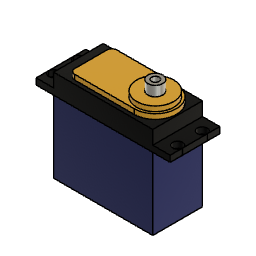
标准舵机 v4 (Autodesk Fusion 360 design; units mm, degrees)
Autodesk Fusion 360 part; units mm, degrees
note: some values were not read from the file. Set by a fixed rule: which sketch regions a step uses.
sketch "草图1" plane through (0, 0, 0) normal (0, 0, 1) x (1, 0, 0)
  line L0 (0, 0) -> (40, 0)
  line L1 (40, 0) -> (40, 20)
  line L2 (40, 20) -> (0, 20)
  line L3 (0, 20) -> (0, 0)
  dimension "d1" = 40
  dimension "d2" = 20
  constraint horizontal L0
  constraint vertical L1
  constraint horizontal L2
  constraint vertical L3
  constraint coincident L0.start L3.end
  measures "d1" distance of L0.start L0.end
  measures "d2" distance of L0.start L2.end
extrude "拉伸1" add sketch "草图1" along normal blind 29 makes body 1
sketch "草图2" plane through (0, 0, 29) normal (0, 0, 1) x (-1, 0, 0)
  line L0 (0, -20) -> (0, 0)
  line L1 (0, 0) -> (-40, 0)
  line L2 (-40, 0) -> (-40, -20)
  line L3 (-40, -20) -> (0, -20)
  line L4 (7, -20) -> (-47, -20)
  line L5 (-47, -20) -> (-47, 0)
  line L6 (-47, 0) -> (7, 0)
  line L7 (7, 0) -> (7, -20)
  line L8 (-20, -21.776) -> (-20, 15.224)
  line L9 (-62, -9.9999) -> (-62, -10)
  line L10 (-62, -10) -> (12.0034, -10)
  line L11 (12.0034, -10) -> (12.0034, -9.9999)
  circle A0 centre (5, -15) radius 2
  circle A1 centre (-45, -15) radius 2
  circle A2 centre (5, -5) radius 2
  circle A3 centre (-45, -5) radius 2
  dimension "d5" = 54
  dimension "d6" = 20
  dimension "d7" = 4
  dimension "d8" = 50
  dimension "d9" = 10
  constraint horizontal L4
  constraint vertical L5
  constraint horizontal L6
  constraint vertical L7
  constraint vertical L8
  constraint symmetric L0 L2 L8
  constraint symmetric L5 L7 L8
  constraint coincident L0.end L6
  constraint horizontal L10
  constraint symmetric L8 A0 A1
  constraint symmetric L10 A0 A2
  constraint symmetric L10 A1 A3
  constraint symmetric L4 L6 L10
  measures "d5" distance of L4.start L4.end
  measures "d6" distance of L4.start L6.end
  measures "d7" diameter of A0
  measures "d8" distance of A0.centre A1.centre
  measures "d9" distance of A0.centre A2.centre
extrude "拉伸2" add sketch "草图2" 1 faces at (13.3333, 13.3333, 29) along normal blind 2.5 separate body on bodies 1 makes body 2
sketch "草图3" plane through (0, 0, 31.5) normal (0, 0, 1) x (-1, 0, 0)
  line L0 (-47, -20) -> (7, -20)
  line L1 (7, -20) -> (7, -15)
  circle A0 centre (5, -15) radius 2
  line L2 (7, -15) -> (7, -5)
  circle A1 centre (5, -5) radius 2
  line L3 (7, -5) -> (7, 0)
  line L4 (7, 0) -> (-47, 0)
  line L5 (-47, 0) -> (-47, -5)
  circle A2 centre (-45, -5) radius 2
  line L6 (-47, -5) -> (-47, -15)
  circle A3 centre (-45, -15) radius 2
  line L7 (-47, -15) -> (-47, -20)
  line L8 (0, 0) -> (-40, 0)
  line L9 (-40, 0) -> (-40, -20)
  line L10 (-40, -20) -> (0, -20)
  line L11 (0, -20) -> (0, 0)
  dimension "d12" = 40
  constraint horizontal L8
  constraint vertical L9
  constraint horizontal L10
  constraint vertical L11
  constraint coincident L0 L9.end
  constraint coincident L8.start L11.end
  measures "d12" distance of L9.end L10.end
extrude "拉伸3" add sketch "草图3" along normal blind 5.5 contours L0 L4 L8 L9 L10 L11 bodies 2
sketch "草图4" plane through (0, 0, 37) normal (0, 0, 1) x (-1, 0, 0)
  line L0 (0, -20) -> (0, 0)
  line L1 (0, 0) -> (-40, 0)
  line L2 (-40, 0) -> (-40, -20)
  line L3 (-40, -20) -> (0, -20)
  line L4 (-47, -5) -> (-47, -15)
  line L5 (-7, -18.5) -> (-31, -18.5)
  line L6 (-31, -1.5) -> (-7, -1.5)
  line L7 (-5, -3.5) -> (-5, -16.5)
  arc A0 (-31, -1.5) -> (-31, -18.5) centre (-31, -10) ccw
  arc A1 (-7, -18.5) -> (-5, -16.5) centre (-7, -16.5) ccw
  arc A2 (-5, -3.5) -> (-7, -1.5) centre (-7, -3.5) ccw
  dimension "d15" = 17
  dimension "d16" = 16
  dimension "d22" = 10
  dimension "d23" = 5
  dimension "d24" = 2
  constraint horizontal L5
  constraint horizontal L6
  constraint vertical L7
  constraint tangent L5 A0
  constraint tangent L6 A0
  constraint tangent L5 A1
  constraint tangent L7 A1
  constraint tangent L6 A2
  constraint tangent L7 A2
  constraint equal A1 A2
  measures "d15" diameter of A0
  measures "d16" distance of A0.centre L4
  measures "d22" distance of L1 A0.centre
  measures "d23" distance of L0 L7
  measures "d24" radius of A1
extrude "拉伸4" add sketch "草图4" along normal blind 2 separate body contours L5 L6 L7 A0 A1 A2 makes body 3
sketch "草图5" plane through (0, 0, 39) normal (0, 0, 1) x (-1, 0, 0)
  circle A0 centre (-31, -10) radius 7.5
  arc A1 (-7, -18.5) -> (-5, -16.5) centre (-7, -16.5) ccw
  line L0 (-5, -16.5) -> (-5, -3.5)
  arc A2 (-5, -3.5) -> (-7, -1.5) centre (-7, -3.5) ccw
  line L1 (-7, -1.5) -> (-31, -1.5)
  arc A3 (-31, -1.5) -> (-31, -18.5) centre (-31, -10) ccw
  line L2 (-31, -18.5) -> (-7, -18.5)
  dimension "d19" = 15
  constraint coincident A0.centre A3.centre
  measures "d19" diameter of A0
extrude "拉伸5" add sketch "草图5" along normal blind 2 contours A0 bodies 3
sketch "草图6" plane through (0, 0, 41) normal (0, 0, 1) x (-1, 0, 0)
  circle A0 centre (-31, -10) radius 7.5
  circle A1 centre (-31, -10) radius 3
  dimension "d25" = 6
  constraint concentric A0 A1
  measures "d25" diameter of A1
extrude "拉伸6" add sketch "草图6" along normal blind 4 separate body contours A1 makes body 4
sketch "草图7" plane through (0, 0, 45) normal (0, 0, 1) x (-1, 0, 0)
  circle A0 centre (-31, -10) radius 3
  circle A1 centre (-31, -10) radius 1.5
  dimension "d28" = 3
  constraint concentric A0 A1
  measures "d28" diameter of A1
extrude "拉伸7" cut sketch "草图7" against normal blind 6 contours A1 bodies 3 4
copy_body "实体->零部件1" bodies 1 removing the originals makes body 5 in component "Component'"
copy_body "实体->零部件2" bodies 2 removing the originals makes body 6 in component "Component''"
copy_body "实体->零部件3" bodies 3 removing the originals makes body 7 in component "Component'''"
copy_body "实体->零部件4" bodies 4 removing the originals makes body 8 in component "Component''''"
component "Component'" placed x (1, 0, 0) y (0, 1, 0) z (0, 0, 1) at (0, 0, 0)
component "Component''" placed x (1, 0, 0) y (0, 1, 0) z (0, 0, 1) at (0, 0, 0)
component "Component'''" placed x (1, 0, 0) y (0, 1, 0) z (0, 0, 1) at (0, 0, 0)
component "Component''''" placed x (1, 0, 0) y (0, 1, 0) z (0, 0, 1) at (0, 0, 0)
